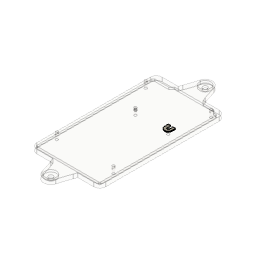
Arduino Mega Mount (Autodesk Fusion 360 design; units mm, degrees)
Autodesk Fusion 360 part; units mm, degrees
sketch "Arduino Mega Sketch" plane through (0, 0, 0) normal (0, 0, 1) x (1, 0, 0) in component "Arduino Mega"
  line L0 (26.13, -50.56) -> (-26.13, -50.56)
  line L1 (-26.63, -50.06) -> (-26.63, 50.56)
  line L2 (-26.63, 50.56) -> (26.63, 50.56)
  line L3 (26.63, 47.56) -> (26.63, -50.06)
  line L4 (26.63, -50.56) -> (-26.63, 50.56) construction
  line L5 (-26.63, -50.56) -> (26.63, 50.56) construction
  line L6 (-13.2245, 50.56) -> (-13.2245, 48.06) construction
  line L7 (-26.63, 48.06) -> (26.63, 48.06)
  line L8 (26.13, 48.06) -> (24.13, 48.06) construction
  line L9 (24.13, 48.06) -> (24.13, 50.56)
  line L10 (-26.63, 48.06) -> (-13.63, 48.06)
  line L11 (-13.63, 48.06) -> (-13.63, 50.56)
  line L12 (-13.63, 48.06) -> (-11.13, 50.56)
  line L13 (-13.63, 48.06) -> (-10.0945, 48.06) construction
  line L14 (24.13, 48.06) -> (21.63, 50.56)
  circle A0 centre (-24.51, 39.61) radius 1.59
  circle A1 centre (24.51, 45.94) radius 1.59
  circle A2 centre (24.51, -36.78) radius 1.59
  circle A3 centre (-24.51, -35.78) radius 1.59
  circle A4 centre (-8.98, 15.3) radius 1.59
  circle A5 centre (18.81, 15.3) radius 1.59
  line L15 (-26.63, 47.0054) -> (-25.5754, 48.06)
  line L16 (-26.63, 47.0054) -> (-25.1385, 47.0054) construction
  arc A6 (26.63, 47.56) -> (26.13, 48.06) centre (26.13, 47.56) ccw
  arc A7 (26.13, -50.56) -> (26.63, -50.06) centre (26.13, -50.06) ccw
  arc A8 (-26.63, -50.06) -> (-26.13, -50.56) centre (-26.13, -50.06) ccw
  dimension "d5" = 53.26
  dimension "d6" = 101.12
  dimension "d7" = 2.5
  dimension "d8" = 2.5
  dimension "d9" = 13
  dimension "d10" = 45
  dimension "d11" = 90
  dimension "d12" = 3.18
  dimension "d13" = 3.18
  dimension "d14" = 3.18
  dimension "d15" = 3.18
  dimension "d16" = 3.18
  dimension "d17" = 3.18
  dimension "d18" = 8.45
  dimension "d19" = 2.12
  dimension "d20" = 2.12
  dimension "d21" = 2.12
  dimension "d22" = 2.12
  dimension "d23" = 2.12
  dimension "d24" = 13.78
  dimension "d25" = 14.78
  dimension "d26" = 7.82
  dimension "d27" = 27.79
  dimension "d28" = 35.26
  dimension "d29" = 35.26
  dimension "d32" = 45
  dimension "d33" = 0.5
  dimension "d34" = 0.5
  dimension "d35" = 0.5
  constraint horizontal L0
  constraint perpendicular L0 L1
  constraint parallel L0 L2
  constraint parallel L1 L3
  constraint coincident L4 origin
  constraint coincident L5 origin
  constraint coincident L2 L6.start
  constraint perpendicular L2 L6
  constraint coincident L1 L7.start
  constraint coincident L3 L7.end
  constraint perpendicular L3 L7
  constraint perpendicular L3 L8
  constraint coincident L2 L9.end
  constraint perpendicular L2 L9
  constraint perpendicular L1 L10
  constraint coincident L2 L11.end
  constraint perpendicular L2 L11
  constraint horizontal L13
  constraint coincident L2 L12.end
  constraint coincident L2 L14.end
  constraint horizontal L16
  constraint coincident L1 L15.start
  constraint coincident L7 L15.end
  constraint coincident L2.end L3
  constraint coincident L7.end L8
  constraint tangent L3 A6
  constraint tangent L8 A6
  constraint coincident L4.start L0
  constraint coincident L4.start L3
  constraint tangent L0 A7
  constraint tangent L3 A7
  constraint coincident L5.start L0
  constraint coincident L5.start L1
  constraint tangent L0 A8
  constraint tangent L1 A8
  measures "d5" distance of L1.end L2.end
  measures "d6" distance of L5.start L1.end
  measures "d7" distance of L6.start L6.end
  measures "d8" distance of L7.end L8.end
  measures "d9" distance of L7.start L10.end
  measures "d10" angle of L12 L13
  measures "d11" angle of L12 L14
  measures "d12" diameter of A0
  measures "d13" diameter of A1
  measures "d14" diameter of A2
  measures "d15" diameter of A3
  measures "d16" diameter of A4
  measures "d17" diameter of A5
  measures "d18" distance of L7 A0.centre
  measures "d19" distance of L1 A0.centre
  measures "d20" distance of L7 A1.centre
  measures "d21" distance of L3 A1.centre
  measures "d22" distance of L3 A2.centre
  measures "d23" distance of L1 A3.centre
  measures "d24" distance of L0 A2.centre
  measures "d25" distance of L0 A3.centre
  measures "d26" distance of L3 A5.centre
  measures "d27" horizontal distance of A4.centre A5.centre
  measures "d28" distance of L2 A5.centre
  measures "d29" distance of L2 A4.centre
  measures "d32" angle of L15 L16
  measures "d33" radius of A6
  measures "d34" radius of A7
  measures "d35" radius of A8
extrude "Extrusion of the Arduino Mega' s body." add sketch "Arduino Mega Sketch" along normal blind 1.6 contours L0 L1 L3 L7 L10 L15 A6 A7 A8 | L2 L7 L12 L14 makes body 1 in component "Arduino Mega"
sketch "Mount sketch" plane through (0, 0, 0) normal (0, 0, 1) x (1, 0, 0) in component "Mount"
  circle A0 centre (18.81, 15.3) radius 1.59
  circle A1 centre (24.51, -36.78) radius 1.59
  circle A2 centre (-24.51, 39.61) radius 1.59
  circle A3 centre (-8.98, 15.3) radius 1.59
  circle A4 centre (-24.51, -35.78) radius 1.59
  circle A5 centre (24.51, 45.94) radius 1.59
  line L0 (-26.63, 47.0054) -> (-26.63, -50.06)
  arc A6 (-26.63, -50.06) -> (-26.13, -50.56) centre (-26.13, -50.06) ccw
  line L1 (-26.13, -50.56) -> (26.13, -50.56)
  arc A7 (26.13, -50.56) -> (26.63, -50.06) centre (26.13, -50.06) ccw
  line L2 (26.63, -50.06) -> (26.63, 47.56)
  arc A8 (26.63, 47.56) -> (26.13, 48.06) centre (26.13, 47.56) ccw
  line L3 (26.13, 48.06) -> (24.13, 48.06)
  line L4 (24.13, 48.06) -> (21.63, 50.56)
  line L5 (21.63, 50.56) -> (-11.13, 50.56)
  line L6 (-11.13, 50.56) -> (-13.63, 48.06)
  line L7 (-13.63, 48.06) -> (-25.5754, 48.06)
  line L8 (-25.5754, 48.06) -> (-26.63, 47.0054)
  line L9 (24.13, 53.06) -> (-24.13, 53.06)
  line L10 (-29.13, 48.06) -> (-29.13, -48.06)
  line L11 (-24.13, -53.06) -> (24.13, -53.06)
  line L12 (29.13, -48.06) -> (29.13, 48.06)
  line L13 (29.13, 53.06) -> (-29.13, -53.06) construction
  line L14 (-29.13, 53.06) -> (29.13, -53.06) construction
  arc A9 (-24.13, 53.06) -> (-29.13, 48.06) centre (-24.13, 48.06) ccw
  arc A10 (29.13, 48.06) -> (24.13, 53.06) centre (24.13, 48.06) ccw
  arc A11 (24.13, -53.06) -> (29.13, -48.06) centre (24.13, -48.06) ccw
  arc A12 (-29.13, -48.06) -> (-24.13, -53.06) centre (-24.13, -48.06) ccw
  circle A13 centre (0, 65.36) radius 1.9
  circle A14 centre (0, 65.36) radius 4.1
  line L15 (0, 1.75) -> (0, 22.5)
  circle A15 centre (0, 65.36) radius 4.7
  line L16 (0, 65.36) -> (-8, 65.36) construction
  line L17 (0, 65.36) -> (8, 65.36) construction
  line L18 (-8, 65.36) -> (5.0894, 65.36) construction
  line L19 (8, 65.36) -> (21.0894, 65.36) construction
  arc A16 (5.9119, 67.0074) -> (-5.9119, 67.0074) centre (0, 65.36) ccw
  line L20 (9.4881, 55.859) -> (10.5069, 53.06)
  line L21 (8, 65.36) -> (21.0894, 65.36) construction
  line L22 (-9.4883, 55.8583) -> (-10.5068, 53.06)
  arc A17 (-9.4883, 55.8583) -> (-5.9119, 67.0074) centre (-151.8517, 107.6744) ccw
  arc A18 (5.9119, 67.0074) -> (9.4881, 55.859) centre (151.8516, 107.675) ccw
  line L23 (20, 0) -> (2.5, 0)
  arc A19 (-5.9119, -67.0074) -> (5.9119, -67.0074) centre (0, -65.36) ccw
  arc A20 (-5.9119, -67.0074) -> (-9.4883, -55.8583) centre (-151.8517, -107.6744) ccw
  line L24 (-9.4883, -55.8583) -> (-10.5068, -53.06)
  arc A21 (9.4881, -55.859) -> (5.9119, -67.0074) centre (151.8516, -107.675) ccw
  line L25 (9.4881, -55.859) -> (10.5069, -53.06)
  circle A22 centre (0, -65.36) radius 4.7
  circle A23 centre (0, -65.36) radius 4.1
  circle A24 centre (0, -65.36) radius 1.9
  line L26 (26.13, 48.36) -> (24.2543, 48.36)
  line L27 (24.2543, 48.36) -> (21.7543, 50.86)
  line L28 (21.7543, 50.86) -> (-11.2543, 50.86)
  line L29 (-11.2543, 50.86) -> (-13.7543, 48.36)
  line L30 (-13.7543, 48.36) -> (-25.6996, 48.36)
  line L31 (-25.6996, 48.36) -> (-26.93, 47.1296)
  line L32 (-26.93, 47.1296) -> (-26.93, -50.06)
  arc A25 (-26.93, -50.06) -> (-26.13, -50.86) centre (-26.13, -50.06) ccw
  line L33 (-26.13, -50.86) -> (26.13, -50.86)
  arc A26 (26.13, -50.86) -> (26.93, -50.06) centre (26.13, -50.06) ccw
  line L34 (26.93, -50.06) -> (26.93, 47.56)
  arc A27 (26.93, 47.56) -> (26.13, 48.36) centre (26.13, 47.56) ccw
  circle A28 centre (-24.51, 39.61) radius 1.09
  circle A29 centre (-24.51, 39.61) radius 0.9
  circle A30 centre (24.51, 45.94) radius 1.09
  circle A31 centre (24.51, 45.94) radius 0.9
  circle A32 centre (18.81, 15.3) radius 1.09
  circle A33 centre (18.81, 15.3) radius 0.9
  circle A34 centre (-8.98, 15.3) radius 1.09
  circle A35 centre (-8.98, 15.3) radius 0.9
  circle A36 centre (-24.51, -35.78) radius 1.09
  circle A37 centre (-24.51, -35.78) radius 0.9
  circle A38 centre (24.51, -36.78) radius 1.09
  circle A39 centre (24.51, -36.78) radius 0.9
  dimension "d36" = 58.26
  dimension "d37" = 106.12
  dimension "d40" = 5
  dimension "d42" = 5
  dimension "d45" = 3.8
  dimension "d46" = 8.2
  dimension "d47" = 12.3
  dimension "d50" = 0.6
  dimension "d51" = 8
  dimension "d52" = 8
  dimension "d55" = 70
  dimension "d56" = 140
  dimension "d57" = 151.5
  dimension "d58" = 0.3
  dimension "d66" = 2.18
  dimension "d67" = 1.8
  dimension "d68" = 2.18
  dimension "d69" = 1.8
  dimension "d70" = 2.18
  dimension "d71" = 1.8
  dimension "d72" = 2.18
  dimension "d73" = 1.8
  dimension "d74" = 2.18
  dimension "d75" = 1.8
  dimension "d76" = 2.18
  dimension "d77" = 1.8
  constraint horizontal L9
  constraint perpendicular L9 L10
  constraint parallel L9 L11
  constraint parallel L10 L12
  constraint coincident L13 origin
  constraint coincident L14 origin
  constraint coincident L14.start L10
  constraint coincident L14.start L9
  constraint tangent L10 A9
  constraint tangent L9 A9
  constraint coincident L13.start L9
  constraint coincident L13.start L12
  constraint tangent L9 A10
  constraint tangent L12 A10
  constraint coincident L14.end L12
  constraint coincident L14.end L11
  constraint tangent L12 A11
  constraint tangent L11 A11
  constraint equal A10 A11
  constraint coincident L13.end L11
  constraint coincident L13.end L10
  constraint tangent L11 A12
  constraint tangent L10 A12
  constraint equal A10 A12
  constraint concentric A13 A14
  constraint coincident A13.centre L15
  constraint coincident A13.centre A14.centre
  constraint horizontal L16
  constraint parallel L16 L17
  constraint horizontal L18
  constraint horizontal L19
  constraint concentric A14 A16
  constraint horizontal L21
  constraint coincident L9 L20.end
  constraint coincident L9 L22.end
  constraint tangent A16 A17
  constraint tangent L22 A17
  constraint tangent A16 A18
  constraint tangent L20 A18
  constraint equal A17 A18
  constraint symmetric A13 L23 A24
  constraint symmetric A14 L23 A23
  constraint symmetric A15 L23 A22
  constraint symmetric A16 L23 A19
  constraint symmetric L20.end L23 L25.end
  constraint symmetric L22.end L23 L24.end
  constraint symmetric L22.start L23 A20.end
  constraint symmetric A16.end L23 A19.start
  constraint symmetric A17 L23 A20
  constraint symmetric L20.start L23 A21.start
  constraint symmetric A16.start L23 A19.end
  constraint symmetric A18 L23 A21
  constraint concentric A2 A28
  constraint concentric A2 A29
  constraint concentric A5 A30
  constraint concentric A30 A31
  constraint concentric A0 A32
  constraint concentric A0 A33
  constraint concentric A3 A34
  constraint concentric A34 A35
  constraint concentric A4 A36
  constraint concentric A36 A37
  constraint concentric A1 A38
  constraint concentric A1 A39
  measures "d36" distance of L13.end L14.end
  measures "d37" distance of L14.start L13.end
  measures "d40" radius of A9
  measures "d42" radius of A10
  measures "d45" diameter of A13
  measures "d46" diameter of A14
  measures "d47" distance of L9 A13.centre
  measures "d51" distance of A13.centre L16.end
  measures "d52" distance of A13.centre L17.end
  measures "d55" angle of L20 L21
  measures "d56" angle of L20 L22
  measures "d57" radius of A17
  measures "d66" diameter of A28
  measures "d67" diameter of A29
  measures "d68" diameter of A30
  measures "d69" diameter of A31
  measures "d70" diameter of A32
  measures "d71" diameter of A33
  measures "d72" diameter of A34
  measures "d73" diameter of A35
  measures "d74" diameter of A36
  measures "d75" diameter of A37
  measures "d76" diameter of A38
  measures "d77" diameter of A39
extrude "Extrusion of the mount's base." add sketch "Mount sketch" along normal blind 1.8 separate body contours A0 | A1 | A2 | A3 | A4 | A5 | L0 A6 L1 A7 L2 A8 L3 L4 L5 L6 L7 L8 | L9 L10 L11 L12 A9 A10 A11 A12 | L9 A16 L20 L22 A17 A18 | L11 A19 A20 L24 A21 L25 | A14 | A15 | A22 | A23 | L26 L27 L28 L29 L30 L31 L32 A25 L33 A26 L34 A27 | A28 | A29 | A30 | A31 | A32 | A33 | A34 | A35 | A36 | A37 | A38 | A39 makes body 2 in component "Mount"
extrude "Extrusion of the mount's walls." add sketch "Mount sketch" along normal blind 1.8 from surface at 1.8 contours L9 L10 L11 L12 A9 A10 A11 A12 | L9 A16 L20 L22 A17 A18 | L11 A19 A20 L24 A21 L25 bodies 2 in component "Mount"
extrude "Extrusion of the Arduino Mega's mount support base." add sketch "Mount sketch" along normal blind 3.6 from surface at 1.8 contours A28 | A29 | A30 | A31 | A32 | A33 | A34 | A35 | A36 | A37 | A38 | A39 bodies 2 in component "Mount"
extrude "Extrusion of the Arduino Mega mount supports inner grove. " add sketch "Mount sketch" along normal blind 1 from surface at 5.4 contours A28 | A29 | A30 | A31 | A33 | A35 | A36 | A37 | A38 | A39 bodies 2 in component "Mount"
extrude "Extrusion of the Arduino Mega mount supports inner grove top. " add sketch "Mount sketch" along normal blind 1.2 from surface at 6.4 contours A28 | A29 | A30 | A31 | A32 | A33 | A34 | A35 | A36 | A37 | A38 | A39 bodies 2 in component "Mount"
ref_plane "WorkPlane1" through (24.51, 47.03, 7.6) normal (0, 1, 0) x (-1, 0, 0) in component "Mount"
sketch "Arduino Mega's mount support cutout circle sketch." plane through (0, 47.03, 0) normal (0, 1, 0) x (1, 0, 0) in component "Mount"
  circle A0 centre (24.51, -6.1) radius 0.5
  line L0 (24.51, 1.1) -> (24.51, -10.5)
  line L1 (23.42, -7.6) -> (25.6, -7.6)
  circle A1 centre (-24.51, -6.1) radius 0.5
  line L2 (-25.6, -7.6) -> (-23.42, -7.6)
  dimension "d88" = 1
  dimension "d89" = 1.5
  dimension "d92" = 1
  dimension "d93" = 1.5
  constraint coincident A0.centre L0
  measures "d88" diameter of A0
  measures "d89" distance of A0.centre L1
  measures "d92" diameter of A1
  measures "d93" distance of A1.centre L2
extrude "Extrusion cutout of the Arduino Mega's mount supports inner hole." cut sketch "Arduino Mega's mount support cutout circle sketch." against normal blind 89 bodies 2 in component "Mount"
sketch "Arduino Mega's mount support clip sketch." plane through (0, 0, 0) normal (0, 0, 1) x (1, 0, 0) in component "Support Clip"
  circle A0 centre (18.81, 15.3) radius 1.09
  circle A1 centre (18.81, 15.3) radius 0.9
  circle A2 centre (18.81, 15.3) radius 1.59
  circle A3 centre (18.81, 15.3) radius 3.0784
  line L0 (15.7316, 18.4479) -> (21.8884, 18.4479)
  line L1 (21.8884, 18.4479) -> (21.8884, 15.3)
  line L2 (15.7316, 15.3) -> (15.7316, 18.4479)
  line L3 (15.7316, 18.4479) -> (21.8884, 12.1521) construction
  line L4 (21.8884, 18.4479) -> (15.7316, 12.1521) construction
  circle A4 centre (18.81, 15.3) radius 1
  line L5 (18.81, 15.3) -> (19.81, 15.3) construction
  line L6 (18.81, 15.3) -> (17.81, 15.3) construction
  line L7 (17.81, 15.3) -> (17.81, 18.4479)
  line L8 (19.81, 15.3) -> (19.81, 18.4479)
  point P0 (18.81, 15.3)
  dimension "d94" = 0.1
  constraint concentric A1 A3
  constraint horizontal L0
  constraint perpendicular L0 L1
  constraint parallel L1 L2
  constraint coincident L3 P0
  constraint coincident L4 P0
  constraint coincident P0 A0.centre
  constraint tangent A3 L2
  constraint coincident A3 L1.end
  constraint coincident A3 L2.start
  constraint coincident A4 L5.end
  constraint horizontal L5
  constraint coincident A4 L6.end
  constraint parallel L5 L6
  constraint coincident L0 L7.end
  constraint perpendicular L0 L7
  constraint coincident L0 L8.end
  constraint perpendicular L0 L8
extrude "Extrusion of the Arduino Mega's mount support inner grove clip." add sketch "Arduino Mega's mount support clip sketch." along normal blind 0.7 separate body contours A0 A4 L7 L8 | A0 A2 L7 L8 | A2 A3 L7 L8 | A3 L0 L1 L8 | A3 L0 L2 L7 picked at (17.7525, 15.3285) picked at (17.4904, 15.8248) picked at (16.2392, 15.1442) makes body 3 in component "Support Clip"
component "Arduino Mega" placed x (1, 0, 0) y (0, 1, 0) z (0, 0, 1) at (0, 0, 0)
component "Mount" placed x (1, 0, 0) y (0, 1, 0) z (0, 0, 1) at (0, 0, 0)
component "Support Clip" placed x (1, 0, 0) y (0, 1, 0) z (0, 0, 1) at (0, 0, 0)
equation "am_length = 101.12 mm" comment "Length of the arduino mega."
equation "am_width = 53.26 mm" comment "Width of the arduino mega."
equation "am_mhole_diam = 3.18 mm" comment "Diameter of the mounting holes on the arduino mega."
equation "am_bthickness = 1.6 mm" comment "Thickness of the board of the arduino mega."
equation "d5 = am_width"
equation "d6 = am_length"
equation "d12 = am_mhole_diam"
equation "d13 = am_mhole_diam"
equation "d14 = am_mhole_diam"
equation "d15 = am_mhole_diam"
equation "d16 = am_mhole_diam"
equation "d17 = am_mhole_diam"
equation "d19 = am_mhole_diam * ( 2 / 3 )"
equation "d20 = am_mhole_diam * ( 2 / 3 )"
equation "d21 = am_mhole_diam * ( 2 / 3 )"
equation "d22 = am_mhole_diam * ( 2 / 3 )"
equation "d23 = am_mhole_diam * ( 2 / 3 )"
equation "d26 = 6.23 mm + ( am_mhole_diam / 2 )"
equation "d30 = am_bthickness"
equation "d36 = am_width + mwall_offset"
equation "d37 = am_length + mwall_offset"
equation "mwall_offset = 5 mm" comment "Offset of the mount from the perimeter of the Arduino Mega."
equation "mwall_thickness = 1.8 mm" comment "Thickness of the mount."
equation "d40 = mwall_fillet"
equation "mwall_fillet = 5 mm" comment "Fillet of the mount wall edges."
equation "d42 = mwall_fillet"
equation "screwh_diam = 8.2 mm" comment "Diameter of the mounting screw head (drywall)."
equation "screwb_diam = 3.8 mm" comment "Diameter of the mounting screw body."
equation "d45 = screwb_diam"
equation "d46 = screwh_diam"
equation "d47 = screwh_diam * 1.5"
equation "s_tolerance = 0.1 mm" comment "Small Tolerance of the 3D printer."
equation "b_tolerance = 0.3 mm" comment "Big tolerance of the 3D printer."
equation "d50 = b_tolerance * 2"
equation "d58 = b_tolerance"
equation "d59 = mwall_thickness"
equation "d61 = mwall_thickness"
equation "d62 = mwall_thickness"
equation "ams_diam = am_mhole_diam - 1 mm" comment "Diameter of the Arduino Mega support on the mount."
equation "amsi_diam = 1.8 mm" comment "Diameter of the Arduino Mega support inner groves on the mount."
equation "d66 = ams_diam"
equation "d67 = amsi_diam"
equation "d68 = ams_diam"
equation "d69 = amsi_diam"
equation "d70 = ams_diam"
equation "d71 = amsi_diam"
equation "d72 = ams_diam"
equation "d73 = amsi_diam"
equation "d74 = ams_diam"
equation "d75 = amsi_diam"
equation "d76 = ams_diam"
equation "d77 = amsi_diam"
equation "d78 = mwall_thickness"
equation "d79 = 2 * mwall_thickness"
equation "d81 = 3 * mwall_thickness"
equation "d84 = 3 * mwall_thickness + 1 mm"
equation "amsi_height = 1 mm" comment "Height of the Arduino Mega's iiner grove support on the mount."
equation "d94 = s_tolerance"
equation "d95 = amsi_height - b_tolerance"
named bodies: "AM Mount"
